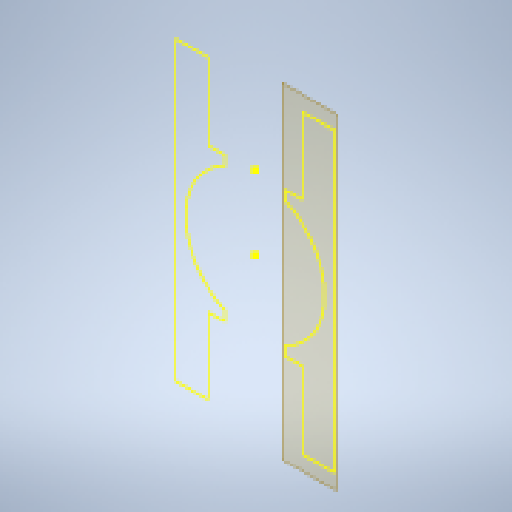
# Autodesk Inventor part: Servo Mount
Saved by Autodesk Inventor 2024 (Build 280153000, 153)
## iProperties
Created: 2024-11-24
Part Number: Servo Mount
Material: Generic
Document SubType Name: Modeling
Designer: Tommy Rohmann
Density: 1 g/cm^3
Appearance: Default
Author: Tommy Rohmann
Autodesk Inventor part; units mm, degrees
ref_plane "YZ Plane" through (0, 0, 0) normal (1, 0, 0) x (0, 1, 0)
ref_plane "XZ Plane" through (0, 0, 0) normal (0, 1, 0) x (-1, 0, 0)
ref_plane "XY Plane" through (0, 0, 0) normal (0, 0, 1) x (1, 0, 0)
ref_plane "Work Plane1" through (0, 0, 0) normal (0, 0, 1) x (1, 0, 0)
sketch "Sketch1" plane through (0, 0, 0) normal (0, 0, 1) x (1, 0, 0)
  line L0 (-7.5184, -0.3239) -> (-7.5184, 11.8935) projected
  line L1 (-12.7635, 11.8935) -> (-7.5184, 11.8935) projected
  line L2 (-12.7635, -35.6806) -> (-12.7635, 11.8935) projected
  line L3 (-12.7635, -35.6806) -> (-7.5184, -35.6806) projected
  line L4 (-7.5184, -23.4632) -> (-7.5184, -35.6806) projected
  line L5 (-4.826, -23.4632) -> (-7.5184, -23.4632) projected
  line L6 (-4.826, -21.9739) -> (-4.826, -23.4632) projected
  arc A0 (-4.826, -1.8132) -> (-4.826, -21.9739) centre (0, -11.8935) ccw projected
  line L7 (-4.826, -1.8132) -> (-4.826, -0.3239) projected
  line L8 (-4.826, -0.3239) -> (-7.5184, -0.3239) projected
  line L9 (7.5184, 11.8935) -> (7.5184, -0.3239) projected
  line L10 (7.5184, -0.3239) -> (4.826, -0.3239) projected
  line L11 (4.826, -0.3239) -> (4.826, -1.8132) projected
  arc A1 (4.826, -21.9739) -> (4.826, -1.8132) centre (0, -11.8935) ccw projected
  line L12 (4.826, -23.4632) -> (4.826, -21.9739) projected
  line L13 (7.5184, -23.4632) -> (4.826, -23.4632) projected
  line L14 (7.5184, -35.6806) -> (7.5184, -23.4632) projected
  line L15 (7.5184, -35.6806) -> (12.7635, -35.6806) projected
  line L16 (12.7635, 11.8935) -> (12.7635, -35.6806) projected
  line L17 (7.5184, 11.8935) -> (12.7635, 11.8935) projected
  circle A2 centre (0, -17.6085) radius 16.891 projected
  line L18 (0, -15.5765) -> (-22.4394, -15.5765) projected
  line L19 (2.032, 11.8935) -> (2.032, -35.6806) projected
  line L20 (0, -11.8935) -> (0, -34.4995)
  line L21 (2.032, -9.8615) -> (-22.606, -9.8616)
  line L22 (12.7635, -35.6806) -> (-22.606, -35.6806)
  line L23 (-22.606, -35.6806) -> (-22.606, 11.8935)
  line L24 (-22.606, 11.8935) -> (-12.7635, 11.8935)
  line L25 (-22.606, -35.6806) -> (15.494, -35.6806)
  line L26 (15.494, -35.6806) -> (15.494, 11.8936)
  line L27 (-22.606, 11.8935) -> (15.494, 11.8935)
  line L28 (15.494, 11.8935) -> (15.494, -35.6806)
  line L29 (15.494, -35.6806) -> (-22.606, -35.6806)
  line L30 (-22.606, -35.6806) -> (-22.606, 11.8935)
  arc A3 (-22.5145, -9.8615) -> (2.032, -34.408) centre (0, -11.8935) ccw
  arc A4 (2.032, -24.4299) -> (-2.032, -24.4299) centre (0, -11.8936) ccw projected
  point P0 (0, 0)
  point P1 (15.494, 11.8936)
  dimension "d0" = 38.1
  constraints: 22 end point, 6 point on line, 5 perpendicular, 3 point on circle, 2 parallel, 1 centre point, 1 coincident, 1 horizontal, 1 vertical, 1 vertical alignment, 1 other
  measures "d0" distance of L22.end L25.end
extrude "Extrusion1" add sketch "Sketch1" along normal blind 25.4 contours L8 A4 A2 L2 L1 L0 | L0 L27 L19 A4 L8 | A4 L19 A2 L7 L8 | L8 L7 A2 A4 | L2 A2 L21 L23 L24 | L27 L9 L10 A4 L19 | A4 L10 L11 A2 L19 | A4 L21 L2 A2 | A2 L7 A0 L21 A4 | L2 L21 A2 | L17 L16 A2 A4 L10 L9 | A2 L19 L21 A0 L7 | A2 L11 A1 L12 L13 A4 L19 | A4 A2 L11 L10 | L27 L26 A2 L16 | A2 A4 L13 L12 A1 L11 | A2 L16 L14 L13 A4 | A2 L26 L16 | A4 L13 L14 A2 L19 | A2 L26 L25 L16 | L16 L15 L14 A2 | A2 L14 L22 L19
body "Solid1"
